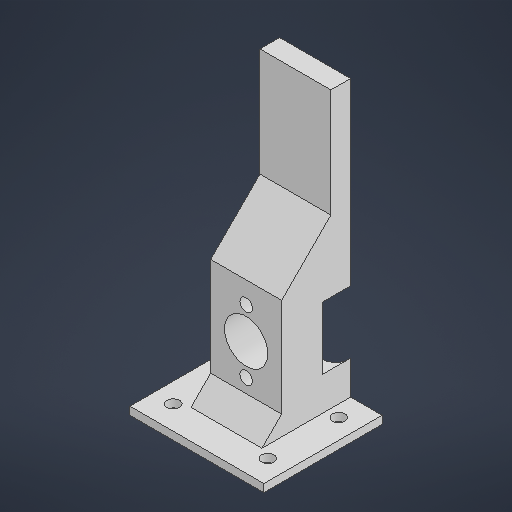
# Autodesk Inventor part: Part6
Saved by Autodesk Inventor 2025.1 (Build 291241000, 241)
## iProperties
Created: 2025-02-22
Part Number: Part6
Material: Generic
Document SubType Name: Modeling
Designer: jerem
Density: 1 g/cm^3
Appearance: Default
Author: jerem
Autodesk Inventor part; units mm, degrees
ref_plane "YZ Plane" through (0, 0, 0) normal (1, 0, 0) x (0, 1, 0)
ref_plane "XZ Plane" through (0, 0, 0) normal (0, 1, 0) x (-1, 0, 0)
ref_plane "XY Plane" through (0, 0, 0) normal (0, 0, 1) x (1, 0, 0)
sketch "Sketch1" plane through (0, 0, 0) normal (0, 1, 0) x (-1, 0, 0)
  line L0 (-17, -15) -> (17, -15)
  line L1 (17, -15) -> (17, 15)
  line L2 (17, 15) -> (-17, 15)
  line L3 (-17, 15) -> (-17, -15)
  line L4 (-17, -15) -> (17, 15) construction
  line L5 (17, -15) -> (-17, 15) construction
  point P0 (0, 0)
  dimension "d0" = 34
  dimension "d1" = 30
  constraints: 12 end point, 2 midpoint, 2 parallel, 1 horizontal, 1 perpendicular
  measures "d0" distance of L2.end L1.end
  measures "d1" distance of L1.end L0.end
extrude "Extrusion1" add sketch "Sketch1" along normal blind 2
sketch "Sketch2" plane through (0, 2, 0) normal (0, 1, 0) x (1, 0, 0)
  line L0 (-17, 15) -> (-17, -15) projected
  line L1 (-17, -15) -> (17, -15) projected
  line L2 (17, -15) -> (17, 15) projected
  line L3 (17, 15) -> (-17, 15) projected
  line L4 (-12, 9) -> (-12, -9) construction
  line L5 (-12, -9) -> (12, -9) construction
  line L6 (12, -9) -> (12, 9) construction
  line L7 (-12, 0) -> (0, 0) construction
  line L8 (0, 0) -> (0, -9) construction
  dimension "d5" = 24
  dimension "d6" = 18
  constraints: 10 end point, 3 parallel, 2 midpoint, 2 perpendicular, 2 vertical
  measures "d5" distance of L4.end L5.end
  measures "d6" distance of L4.start L4.end
hole "Hole1" at (-12, 2, -9) at (-12, 2, 9) at (12, 2, 9) at (12, 2, -9) direction (0, -1, 0) diameter 3.2 end through all
sketch "Sketch3" plane through (0, 2, 0) normal (0, 1, 0) x (1, 0, 0)
  circle A0 centre (12, 9) radius 1.6 projected
  circle A1 centre (12, -9) radius 1.6 projected
  circle A2 centre (-12, -9) radius 1.6 projected
  circle A3 centre (-12, 9) radius 1.6 projected
  line L0 (-17, 15) -> (-17, -15) projected
  line L1 (-17, -15) -> (17, -15) projected
  line L2 (17, -15) -> (17, 15) projected
  line L3 (17, 15) -> (-17, 15) projected
  line L4 (-17, -2.5) -> (17, -2.5)
  circle A4 centre (-12, 9) radius 3
  circle A5 centre (12, 9) radius 3
  line L5 (-9, 15) -> (-9, -15)
  line L6 (9, 15) -> (9, -15)
  point P0 (0, 0)
  point P1 (9, -2.5)
  point P2 (-9, -2.5)
  dimension "d14" = 17.5
  dimension "d15" = 6
  dimension "d16" = 8
  dimension "d17" = 8
  constraints: 6 end point, 6 point on line, 3 perpendicular, 2 centre point, 2 coincident, 1 equal radius
  measures "d14" distance between parallel lines of L4 L3
  measures "d15" diameter of A4
  measures "d16" distance between parallel lines of L0 L5
  measures "d17" distance between parallel lines of L2 L6
extrude "Extrusion2" add sketch "Sketch3" along normal blind 30 contours L3 L6 L4 L5
sketch "Sketch4" plane through (17, 0, -15) normal (0, 0, -1) x (-1, 0, 0)
  line L0 (0, 0) -> (34, 0) projected
  line L1 (34, 0) -> (34, 2) projected
  line L2 (26, 2) -> (34, 2) projected
  line L3 (26, 2) -> (26, 32) projected
  line L4 (8, 32) -> (26, 32) projected
  line L5 (8, 2) -> (8, 32) projected
  line L6 (0, 2) -> (8, 2) projected
  line L7 (0, 0) -> (0, 2) projected
  circle A0 centre (17, 18.5) radius 5.5
  line L8 (17, 18.5) -> (17, 0) construction
  circle A1 centre (17, 18.5) radius 12
  line L9 (17, 18.5) -> (17, 26.5) construction
  circle A2 centre (17, 10.5) radius 1.6
  circle A3 centre (17, 26.5) radius 1.6
  point P0 (26, 26.4373)
  point P1 (8, 26.4373)
  point P2 (8, 10.5627)
  point P3 (26, 10.5627)
  dimension "d20" = 18.5
  dimension "d21" = 24
  dimension "d22" = 11
  dimension "d24" = 8
  dimension "d29" = 3.2
  dimension "d30" = 8
  constraints: 4 centre point, 4 end point, 2 coincident, 1 equal radius, 1 perpendicular, 1 point on line, 1 vertical
  measures "d20" distance of L8.start L8.end
  measures "d21" diameter of A1
  measures "d22" diameter of A0
  measures "d24" distance of L8.start L9.end
  measures "d29" diameter of A2
  measures "d30" distance of L8.start A2.centre
extrude "Extrusion3" cut sketch "Sketch4" against normal blind 7.25 contours L5 A1 L3 | A0 | A2 | A3
extrude "Extrusion4" cut sketch "Sketch4" against normal through all contours A0 | A2 | A3
sketch "Sketch6" plane through (0, 32, 0) normal (0, 1, 0) x (1, 0, 0)
  line L0 (9, 15) -> (-9, 15) projected
  line L1 (-9, 15) -> (-9, -2.5) projected
  line L2 (-9, -2.5) -> (9, -2.5) projected
  line L3 (9, -2.5) -> (9, 15) projected
  line L4 (-9, 10) -> (9, 10)
  point P0 (0, 0)
  dimension "d33" = 5
  constraints: 2 end point, 2 point on line, 1 perpendicular
  measures "d33" distance between parallel lines of L0 L4
extrude "Extrusion6" add sketch "Sketch6" along normal blind 40 contours L3 L4 L1 L0
chamfer "Chamfer1" distance 12.5 angle 45 1 edges at (0, 32, -10)
chamfer "Chamfer2" distance 5 angle 45 1 edges at (0, 2, 2.5)
equation "\"d17\" = d16"
equation "\"d24\" = d30"
body "Solid1"
